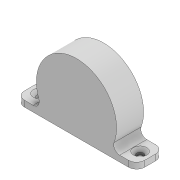
# Autodesk Inventor part: корпус подшипник
Saved by Autodesk Inventor 2021 (Build 250183000, 183)
## iProperties
Created: 2023-02-20
Part Number: корпус подшипник
Material: Типовые
Document SubType Name: Modeling
Designer: Tasya
Density: 1 g/cm^3
Appearance: По умолчанию
Author: Tasya
Autodesk Inventor part; units mm, degrees
ref_plane "YZ Plane" through (0, 0, 0) normal (1, 0, 0) x (0, 1, 0)
ref_plane "XZ Plane" through (0, 0, 0) normal (0, 1, 0) x (-1, 0, 0)
ref_plane "XY Plane" through (0, 0, 0) normal (0, 0, 1) x (1, 0, 0)
sketch "Эскиз1" plane through (0, 0, 0) normal (0, 0, 1) x (1, 0, 0)
  line L0 (-30, 0) -> (30, 0)
  line L1 (-30, 0) -> (-30, 3)
  line L2 (-30, 3) -> (-16.7033, 3)
  line L3 (16.7033, 3) -> (30, 3)
  line L4 (30, 3) -> (30, 0)
  line L5 (0, 0) -> (0, -12) construction
  circle A0 centre (0, 14) radius 11 construction
  circle A1 centre (0, 14) radius 11
  arc A2 (16.7033, 3) -> (-16.7033, 3) centre (0, 14) ccw
  point P0 (0, 3)
  point P1 (0, 46)
  point P2 (0, 25)
  dimension "d3" = 3
  dimension "d8" = 22
  dimension "d9" = 14
  dimension "d25" = 40
  dimension "d39" = 30
  constraints: 12 end point, 4 point on circle, 3 horizontal, 2 centre point, 2 coincident, 1 collinear, 1 midpoint, 1 perpendicular, 1 point on line, 1 vertical, 1 vertical alignment, 3 other
  measures "d3" distance of L0.start L1.end
  measures "d8" diameter of A0
  measures "d9" distance of L5.start A0.centre
  measures "d25" diameter of A2
  measures "d39" distance between parallel lines of L5 L1
extrude "Выдавливание1" add sketch "Эскиз1" along normal blind 10.5
sketch "Эскиз2" plane through (0, 0, 10.5) normal (0, 0, 1) x (1, 0, 0)
  line L0 (-30, 0) -> (30, 0) projected
  line L1 (30, 0) -> (30, 3) projected
  line L2 (30, 3) -> (16.7033, 3) projected
  line L3 (-16.7033, 3) -> (-30, 3) projected
  line L4 (-30, 3) -> (-30, 0) projected
  circle A0 centre (0, 14) radius 11 projected
  arc A1 (16.7033, 3) -> (-16.7033, 3) centre (0, 14) ccw projected
  point P0 (0, 0)
extrude "Выдавливание2" add sketch "Эскиз2" along normal blind 3 contours L4 L3 A1 L2 L1 L0 | A0
fillet "Сопряжение1" radius 4 4 edges at (30, 1.5, 0) (30, 1.5, 13.5) (-30, 1.5, 0) (-30, 1.5, 13.5)
fillet "Сопряжение1" radius 3 2 edges at (16.7033, 3, 6.75) (-16.7033, 3, 6.75)
sketch "Эскиз4" plane through (21.5639, 3, 0) normal (0, 1, 0) x (1, 0, 0)
  line L0 (-43.1277, 0) -> (-43.1277, -13.5) projected
  line L1 (-43.1277, 0) -> (-47.5639, 0) projected
  arc A0 (-47.5639, 0) -> (-51.5639, -4) centre (-47.5639, -4) ccw projected
  line L2 (-51.5639, -4) -> (-51.5639, -9.5) projected
  arc A1 (-51.5639, -9.5) -> (-47.5639, -13.5) centre (-47.5639, -9.5) ccw projected
  line L3 (-43.1277, -13.5) -> (-47.5639, -13.5) projected
  point P0 (-21.5639, 0)
  point P1 (-46.5639, -6.75)
  dimension "d29" = 5
  dimension "d30" = 6.75
  measures "d29" distance from line of L2 point (-46.564, -6.75)
  measures "d30" distance from line of L1 point (-46.564, -6.75)
hole "Отверстие2" at (-25, 3, 6.75) direction (0, -1, 0) diameter 3.4 depth 3.7 countersink diameter 6.6 countersink angle 90 clearance for "с потайной головкой ГОСТ 12876-67" size "M3" standard "ГОСТ"
mirror "Зеркальное отражение2" about plane through (0, 0, 0) normal (1, 0, 0) of "Отверстие2"
